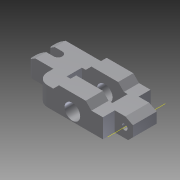
# Autodesk Inventor part: idler mount
Saved by Autodesk Inventor 2012 (Build 160160000, 160)
## iProperties
Created: 2012-01-05
Part Number: idler mount
Material: Default
Document SubType Name: Modeling
Designer: Kennell
Density: 1 g/cm^3
Author: Kennell
Autodesk Inventor part; units mm, degrees
ref_plane "YZ Plane" through (0, 0, 0) normal (1, 0, 0) x (0, 1, 0)
ref_plane "XZ Plane" through (0, 0, 0) normal (0, 1, 0) x (-1, 0, 0)
ref_plane "XY Plane" through (0, 0, 0) normal (0, 0, 1) x (1, 0, 0)
sketch "Sketch1" plane through (0, 0, 0) normal (0, 0, 1) x (1, 0, 0)
  line L0 (0, 0) -> (0, 25)
  line L1 (0, 25) -> (35, 25)
  line L2 (35, 25) -> (35, 18.75)
  line L3 (35, 18.75) -> (44.5, 18.75)
  line L4 (44.5, 18.75) -> (44.5, 6.25)
  line L5 (44.5, 6.25) -> (35, 6.25)
  line L6 (35, 6.25) -> (35, 0)
  line L7 (35, 0) -> (0, 0)
  point P0 (0, 12.5)
  point P1 (44.5, 12.5)
  dimension "d0" = 25
  dimension "d1" = 35
  dimension "d2" = 12.5
  dimension "d3" = 6.25
  dimension "d4" = 9.5
  constraints: 16 end point, 6 parallel, 2 midpoint, 1 collinear, 1 horizontal alignment, 1 perpendicular, 1 vertical
  measures "d0" distance of L0.start L0.end
  measures "d1" distance of L6.end L0.start
  measures "d2" distance of L3.end L4.end
  measures "d3" distance of L5.end L6.end
  measures "d4" distance of L2.end L3.end
extrude "Extrusion1" add sketch "Sketch1" along normal blind 10
hole "Hole1" at (40.2, 6.25, 5) direction (0, 1, 0) diameter 3 end through all
chamfer "Chamfer1" distance 2.5 angle 45 1 edges at (44.5, 12.5, 0)
hole "Hole2" at (19, 0, 4.51) direction (0, 1, 0) diameter 8.2 end through all
sketch "Sketch2" plane through (0, 0, 10) normal (0, 0, 1) x (1, 0, 0)
  line L0 (0, 25) -> (35, 25) projected
  line L1 (35, 0) -> (0, 0) projected
  line L2 (23.1, 25) -> (23.1, 0) projected
  line L3 (14.9, 25) -> (14.9, 0) projected
  line L4 (9, 0) -> (29, 0)
  line L5 (29, 0) -> (29, 25)
  line L6 (29, 25) -> (9, 25)
  line L7 (9, 25) -> (9, 0)
  dimension "d28" = 20
  dimension "d29" = 6
  constraints: 8 end point, 2 parallel, 2 point on line, 1 horizontal, 1 perpendicular
  measures "d28" distance between parallel lines of L5 L7
  measures "d29" distance of L4.end L1.start
extrude "Extrusion2" add sketch "Sketch2" along normal blind 3
chamfer "Chamfer2" distance 3 angle 45 2 edges at (29, 12.5, 13) (9, 12.5, 13)
sketch "Sketch3" plane through (0, 0, 0) normal (-1, 0, 0) x (0, 0, 1)
  line L0 (10, 0) -> (10, 25) projected
  line L1 (0, 25) -> (10, 25)
  line L2 (10, 25) -> (10, 9)
  line L3 (10, 9) -> (0, 9)
  line L4 (0, 9) -> (0, 25)
  dimension "d35" = 16
  constraints: 8 end point, 2 parallel, 1 horizontal, 1 perpendicular, 1 point on line
  measures "d35" distance of L1.end L2.end
extrude "Extrusion3" add sketch "Sketch3" along normal blind 13
hole "Hole3" at (-5.5, 17, 10) direction (0, 0, -1) diameter 4.5 end through all
sketch "Sketch4" plane through (0, 0, 10) normal (0, 0, 1) x (1, 0, 0)
  circle A0 centre (-5.5, 17) radius 2.25 projected
  line L0 (-13, 25) -> (-13, 9) projected
  line L1 (-5.5, 19.25) -> (-13, 19.25)
  line L2 (-13, 19.25) -> (-13, 14.75)
  line L3 (-13, 14.75) -> (-5.5, 14.75)
  line L4 (-5.5, 14.75) -> (-5.5, 19.25)
  constraints: 8 end point, 3 horizontal, 2 parallel, 1 perpendicular, 1 point on line, 1 vertical alignment, 1 other
extrude "Extrusion4" cut sketch "Sketch4" against normal through all contours L4 A0 | A0 L3 L0 L1 picked at (-6.2445, 17.0904)
fillet "Fillet1" radius 2 4 edges at (-13, 25, 5) (-13, 19.25, 5) (-13, 14.75, 5) (-13, 9, 5)
sketch "Sketch5" plane through (0, 9, 0) normal (0, -1, 0) x (1, 0, 0)
  line L0 (0, 10) -> (-11, 10) projected
  line L1 (-13, 10) -> (-13, 0) projected
  line L2 (-13, 10) -> (-11, 10) projected
  line L3 (-13, 10) -> (-9.4444, 10)
  line L4 (-13, 7.7985) -> (-13, 10)
  line L5 (-13, 7.7985) -> (-9.4444, 10)
  dimension "d52" = 3.5556
  dimension "d53" = 2.2015
  constraints: 6 end point, 2 point on line, 1 collinear
  measures "d52" distance of L3.end L1.start
  measures "d53" distance of L4.start L1.start
extrude "Extrusion5" cut sketch "Sketch5" against normal through all
fillet "Fillet2" radius 6 1 edges at (0, 0, 5)
sketch "Sketch6" plane through (0, 0, 13) normal (0, 0, 1) x (1, 0, 0)
  line L0 (9, 0) -> (9, 25) projected
  line L1 (-9.4444, 25) -> (9, 25) projected
  line L2 (12, 25) -> (9, 25) projected
  line L3 (29, 25) -> (26, 25) projected
  line L4 (29, 25) -> (35, 25) projected
  line L5 (9, 0) -> (6, 0) projected
  line L6 (26, 0) -> (29, 0) projected
  line L7 (35, 0) -> (29, 0) projected
  line L8 (23.1, 25) -> (23.1, 0) projected
  line L9 (14.9, 25) -> (14.9, 0) projected
  line L10 (7, 9) -> (31, 9)
  line L11 (31, 9) -> (31, 17)
  line L12 (31, 17) -> (7, 17)
  line L13 (7, 17) -> (7, 9)
  point P0 (0, 0)
  dimension "d55" = 24
  dimension "d56" = 8
  dimension "d57" = 9
  dimension "d58" = 7.9
  constraints: 8 end point, 2 parallel, 1 horizontal, 1 perpendicular
  measures "d55" distance of L12.end L11.end
  measures "d56" distance of L11.end L10.end
  measures "d57" distance between parallel lines of L10 L5
  measures "d58" distance from line of L10.end L8
extrude "Extrusion6" cut sketch "Sketch6" against normal through all
chamfer "Chamfer3" distance 2 distance2 4 1 edges at (44.5, 12.5, 10) measured on face at (44.5, 14.5833, 5)
body "Solid1"
